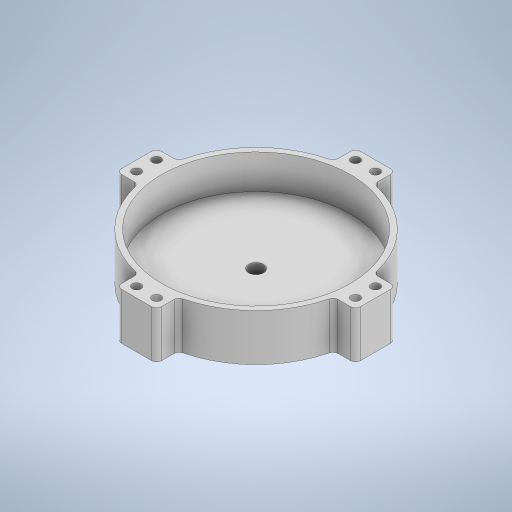
# Autodesk Inventor part: RingCase
Saved by Autodesk Inventor 2023 (Build 270158000, 158)
## iProperties
Created: 2024-01-10
Part Number: RingCase
Material: Generic
Document SubType Name: Modeling
Designer: thesl
Density: 1 g/cm^3
Appearance: Default
Author: thesl
## iProperties of the stored document RingCase_3DPrint.ipt
Created: 2024-01-11
Part Number: RingCase_3DPrint
Material: Generic
Document SubType Name: Modeling
Designer: thesl
Density: 1 g/cm^3
Appearance: Default
Author: thesl
Autodesk Inventor part; units mm, degrees
ref_plane "YZ Plane" through (0, 0, 0) normal (1, 0, 0) x (0, 1, 0)
ref_plane "XZ Plane" through (0, 0, 0) normal (0, 1, 0) x (-1, 0, 0)
ref_plane "XY Plane" through (0, 0, 0) normal (0, 0, 1) x (1, 0, 0)
sketch "Sketch1" plane through (0, 0, 0) normal (0, 1, 0) x (-1, 0, 0)
  circle A0 centre (0, 0) radius 50.8
  circle A1 centre (0, 0) radius 3.81
  dimension "d0" = 101.6
  dimension "d1" = 7.62
  constraints: 2 centre point, 2 coincident
  measures "d0" diameter of A0
  measures "d1" diameter of A1
extrude "Extrusion1" add sketch "Sketch1" along normal blind 6.35
sketch "Sketch2" plane through (0, 6.35, 0) normal (0, 1, 0) x (1, 0, 0)
  circle A0 centre (0, 0) radius 3.81 projected
  circle A1 centre (0, 0) radius 50.8
  circle A2 centre (0, 0) radius 48.006
  dimension "d4" = 96.012
  constraints: 2 centre point, 2 coincident
  measures "d4" diameter of A2
extrude "Extrusion2" add sketch "Sketch2" along normal blind 17.4498 contours A1
fillet "Fillet1" [suppressed]
sketch "Sketch3" plane through (0, 23.7998, 0) normal (0, 1, 0) x (1, 0, 0)
  circle A0 centre (0, 0) radius 48.006 projected
  line L0 (0, 48.006) -> (10.16, 48.006)
  line L1 (10.16, 48.006) -> (10.16, 60.706)
  line L2 (10.16, 60.706) -> (0, 60.706)
  line L3 (0, 60.706) -> (0, 55.6155)
  line L4 (0, 48.006) -> (-10.16, 48.006)
  line L5 (-10.16, 48.006) -> (-10.16, 60.706)
  line L6 (-10.16, 60.706) -> (0, 60.706)
  line L7 (0, 60.706) -> (0, 55.6155)
  line L8 (-55.6768, 0) -> (-60.7568, 0)
  line L9 (-60.7568, 0) -> (-60.7568, 10.16)
  line L10 (-60.7568, 10.16) -> (-48.0568, 10.16)
  line L11 (-48.0568, 10.16) -> (-48.0568, 0)
  line L12 (-55.6768, 0) -> (-60.7568, 0)
  line L13 (-60.7568, 0) -> (-60.7568, -10.16)
  line L14 (-60.7568, -10.16) -> (-48.0568, -10.16)
  line L15 (-48.0568, -10.16) -> (-48.0568, 0)
  line L16 (0, -48.006) -> (10.16, -48.006)
  line L17 (10.16, -48.006) -> (10.16, -60.706)
  line L18 (10.16, -60.706) -> (0, -60.706)
  line L19 (0, -60.706) -> (0, -55.626)
  line L20 (0, -48.006) -> (-10.16, -48.006)
  line L21 (-10.16, -48.006) -> (-10.16, -60.706)
  line L22 (-10.16, -60.706) -> (0, -60.706)
  line L23 (0, -60.706) -> (0, -55.626)
  line L24 (48.006, 0) -> (55.626, 0)
  line L25 (60.706, 0) -> (60.706, 10.16)
  line L26 (60.706, 10.16) -> (48.006, 10.16)
  line L27 (48.006, 10.16) -> (48.006, 0)
  line L28 (48.006, 0) -> (55.626, 0)
  line L29 (60.706, 0) -> (60.706, -10.16)
  line L30 (60.706, -10.16) -> (48.006, -10.16)
  line L31 (48.006, -10.16) -> (48.006, 0)
  line L32 (5.08, -60.706) -> (5.08, -57.8739)
  line L33 (60.706, -5.08) -> (57.8739, -5.08)
  line L34 (-60.7568, -5.08) -> (-57.9247, -5.08)
  line L35 (-5.08, 60.706) -> (-5.08, 55.6155)
  circle A1 centre (-5.08, 55.6155) radius 2.2479
  circle A2 centre (5.08, 55.6155) radius 2.2479
  circle A3 centre (55.626, 5.08) radius 2.2479
  circle A4 centre (55.626, -5.08) radius 2.2479
  circle A5 centre (5.08, -55.626) radius 2.2479
  circle A6 centre (-5.08, -55.626) radius 2.2479
  circle A7 centre (-55.6768, 5.08) radius 2.2479
  circle A8 centre (-55.6768, -5.08) radius 2.2479
  line L36 (-55.6768, -5.08) -> (-55.6768, -2.8321)
  line L37 (-55.6768, 2.8321) -> (-55.6768, 5.08)
  line L38 (0, 55.6155) -> (5.08, 55.6155)
  line L39 (55.626, -5.08) -> (55.626, -2.8321)
  line L40 (55.626, 2.8321) -> (55.626, 5.08)
  line L41 (5.08, -55.626) -> (2.8321, -55.626)
  line L42 (0, -55.626) -> (-5.08, -55.626)
  point P0 (0, -60.706)
  dimension "d25" = 4.4958
  dimension "d29" = 4.4958
  dimension "d8" = 10.16
  dimension "d9" = 12.7
  dimension "d10" = 12.7
  dimension "d11" = 10.16
  dimension "d12" = 10.16
  dimension "d13" = 10.16
  dimension "d14" = 12.7
  dimension "d15" = 10.16
  dimension "d16" = 10.16
  dimension "d17" = 12.7
  dimension "d18" = 10.16
  dimension "d19" = 10.16
  dimension "d20" = 5.08
  dimension "d21" = 5.08
  dimension "d22" = 5.08
  dimension "d23" = 4.4958
  dimension "d24" = 4.4958
  dimension "d26" = 4.4958
  dimension "d27" = 4.4958
  dimension "d28" = 4.4958
  dimension "d30" = 4.4958
  constraints: 86 end point, 16 parallel, 15 perpendicular, 10 horizontal, 9 point on circle, 8 coincident, 6 centre point, 4 point on line, 3 midpoint, 2 vertical, 2 vertical alignment, 4 other
  measures "d8" distance of L2.end L1.end
  measures "d9" distance of L9.end L10.end
  measures "d10" distance of L29.end L30.end
  measures "d11" distance of L29.start L29.end
  measures "d12" distance of L25.start L25.end
  measures "d13" distance of L5.end L6.end
  measures "d14" distance of L0.end L1.end
  measures "d15" distance of L8.end L9.end
  measures "d16" distance of L12.end L13.end
  measures "d17" distance of L16.end L17.end
  measures "d18" distance of L17.end L18.end
  measures "d19" distance of L21.end L22.end
  measures "d20" distance of L32.start L41.start
  measures "d21" distance of L33.start L39.start
  measures "d22" distance of L34.start L36.start
  measures "d23" diameter of A1
  measures "d24" diameter of A2
  measures "d26" diameter of A4
  measures "d27" diameter of A5
  measures "d28" diameter of A6
  measures "d30" diameter of A8
extrude "Extrusion3" add sketch "Sketch3" against normal up to surface (23.7998 mm away) contours L16 L17 L18 L22 L21 L20 | L4 L5 L6 L2 L1 L0 | L27 L26 L25 L29 L30 L31 | L9 L10 L11 L15 L14 L13
fillet "Fillet2" radius 2.54 16 edges at (-49.7736, 11.8999, 10.16) (-60.7568, 11.8999, 10.16) (-60.7568, 11.8999, -10.16) (-49.7736, 11.8999, -10.16) (-10.16, 11.8999, -49.7736) (-10.16, 11.8999, -60.706) (10.16, 11.8999, -60.706) (10.16, 11.8999, -49.7736) (49.7736, 11.8999, -10.16) (60.706, 11.8999, -10.16) (60.706, 11.8999, 10.16) (49.7736, 11.8999, 10.16) (10.16, 11.8999, 49.7736) (10.16, 11.8999, 60.706) (-10.16, 11.8999, 60.706) (-10.16, 11.8999, 49.7736)
body "Solid1"
